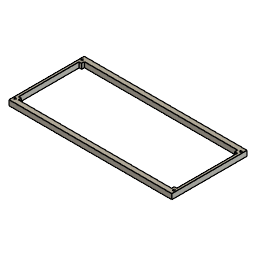
3d printed walls (Autodesk Fusion 360 design; units mm, degrees)
Autodesk Fusion 360 part; units mm, degrees
note: some values were not read from the file. Set by a fixed rule: which face or edge a step refers to.
sketch "Sketch1" plane through (0, 0, 0) normal (0, 1, 0) x (1, 0, 0)
  line L0 (-107.4349, 34.7679) -> (245.6251, 34.7679)
  line L1 (245.6251, 34.7679) -> (245.6251, -118.2321)
  line L2 (245.6251, -118.2321) -> (-107.4349, -118.2321)
  line L3 (-107.4349, -118.2321) -> (-107.4349, 34.7679)
  line L4 (-107.4349, 34.7679) -> (245.6251, 34.7679)
  line L5 (245.6251, 34.7679) -> (245.6251, 29.7679)
  line L6 (-107.4349, 29.7679) -> (-107.4349, 34.7679)
  line L7 (245.6251, 34.7679) -> (240.6251, 34.7679)
  line L8 (157.6216, -118.2321) -> (245.6251, -118.2321)
  line L9 (245.6251, -118.2321) -> (245.6251, 34.7679)
  line L10 (245.6251, -118.2321) -> (-107.4349, -118.2321)
  line L11 (-107.4349, -118.2321) -> (-107.4349, -113.2321)
  line L12 (245.6251, -113.2321) -> (245.6251, -118.2321)
  line L13 (-107.4349, -118.2321) -> (-30.4984, -118.2321)
  line L14 (-102.4349, 34.7679) -> (-107.4349, 34.7679)
  line L15 (-107.4349, 34.7679) -> (-107.4349, -118.2321)
  line L16 (-107.4349, -118.2321) -> (-24.9576, -118.2321)
  line L17 (-96.894, -113.2321) -> (-96.894, -107.2397)
  line L18 (-96.894, -107.2397) -> (-102.4349, -107.2397)
  line L19 (-107.4349, -107.2397) -> (-107.4349, -118.2321)
  circle A0 centre (-103.1349, -114.3777) radius 2.1
  line L20 (-106.1349, -119.3752) -> (-99.8349, -119.3752)
  line L21 (69.0951, -118.2321) -> (69.0951, 34.7679) construction
  line L22 (245.6251, -41.7321) -> (-107.4349, -41.7321) construction
  line L23 (235.0843, -113.2321) -> (235.0843, -107.2397)
  line L24 (235.0843, -107.2397) -> (240.6251, -107.2397)
  circle A1 centre (241.3251, -114.3777) radius 2.1
  line L25 (-96.894, -113.2321) -> (235.0843, -113.2321)
  circle A2 centre (-103.1349, 30.9136) radius 2.1
  line L26 (-96.894, 29.7679) -> (-96.894, 23.7756)
  line L27 (-96.894, 23.7756) -> (-102.4349, 23.7756)
  line L28 (235.0843, 23.7756) -> (240.6251, 23.7756)
  line L29 (235.0843, 29.7679) -> (235.0843, 23.7756)
  circle A3 centre (241.3251, 30.9136) radius 2.1
  line L30 (240.6251, 23.7756) -> (240.6251, -107.2397)
  line L31 (235.0843, 29.7679) -> (-96.894, 29.7679)
  line L32 (-102.4349, -107.2397) -> (-102.4349, 23.7756)
  dimension "d1" = 153
  dimension "d2" = 353.06
  dimension "d3" = 5
  dimension "d4" = 5
  dimension "d5" = 5
  dimension "d6" = 5
  dimension "d8" = 4.2
  dimension "d9" = 4.3
  dimension "d10" = 6.3
  dimension "d11" = 1.3
  dimension "d14" = 3.8543
  dimension "d15" = 10.5408
  dimension "d16" = 10.9923
  dimension "d17" = 5
  dimension "d18" = 5
  dimension "d19" = 5
  constraint horizontal L0
  constraint vertical L1
  constraint horizontal L2
  constraint vertical L3
  constraint horizontal L4
  constraint vertical L5
  constraint vertical L6
  constraint coincident L1 L5.end
  constraint horizontal L7
  constraint horizontal L8
  constraint vertical L9
  constraint coincident L2 L8.start
  constraint horizontal L10
  constraint vertical L11
  constraint vertical L12
  constraint coincident L3 L11.end
  constraint horizontal L13
  constraint horizontal L14
  constraint vertical L15
  constraint coincident L4 L14.start
  constraint horizontal L16
  constraint vertical L17
  constraint horizontal L18
  constraint vertical L19
  constraint perpendicular L19 L20
  constraint midpoint L10 L21.start
  constraint midpoint L4 L21.end
  constraint midpoint L9 L22.start
  constraint midpoint L15 L22.end
  constraint symmetric L17.end L21 L23.end
  constraint symmetric A0 L21 A1
  constraint symmetric L17.end L22 L26.end
  constraint symmetric A0 L22 A2
  constraint symmetric L18.end L22 L27.end
  constraint symmetric L17.start L22 L26.start
  constraint symmetric L22 L23.end L28.start
  constraint symmetric L22 A1 A3
  constraint symmetric L22 L24.end L28.end
  constraint symmetric L22 L23.start L29.start
  measures "d1" distance of L0.start L2.end
  measures "d2" distance of L0.start L0.end
  measures "d3" distance of L14.start L0.start
  measures "d4" distance of L0.end L7.end
  measures "d5" distance of L0.start L6.start
  measures "d6" distance of L2.end L11.end
  measures "d8" diameter of A0
  measures "d9" distance of L3 A0.centre
  measures "d10" distance of L20.start L20.end
  measures "d11" horizontal distance of L2.end L20.start
  measures "d14" distance of L0 A3.centre
  measures "d15" distance of L15 L17
  measures "d16" distance of L10 L18
  measures "d17" distance of L3 L32
  measures "d18" distance of L1 L30
  measures "d19" distance of L2 L25
extrude "Extrude1" add sketch "Sketch1" along normal blind 11.43
extrude "Extrude2" add 4 faces at (216.2906, 3.81, 118.2321) (96.7618, 3.81, 118.2321) (-26.8045, 3.81, 118.2321) (-56.1439, 3.81, 118.2321) along direction (0, 0, 1) blind 5.08
extrude "Extrude3" add 1 faces at (127.9385, 7.62, -34.7679) along direction (0, 0, -1) blind 5.08
equation "d9 = 1.8 mm + 2.5 mm"
